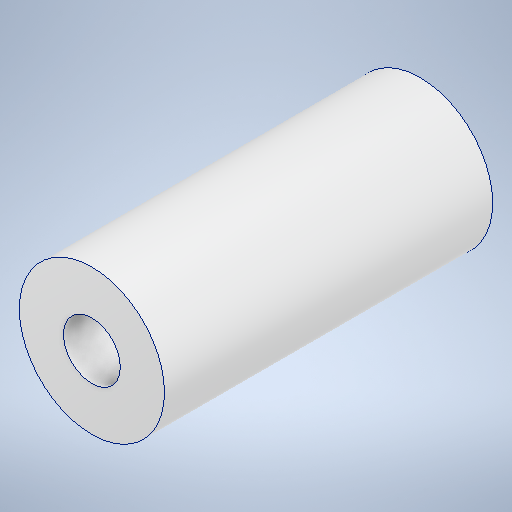
# Autodesk Inventor part: 10-32 0.5 1.131 Inch Stand Off
Saved by Autodesk Inventor 2025.1 (Build 291241020, 241B)
## iProperties
Created: 2024-10-06
Part Number: 10-32 0.5 1.131 Inch Stand Off
Material: Aluminum 6061
Document SubType Name: Modeling
Designer: xmand
Density: 2.7 g/cm^3
Appearance: Aluminum - Flat
Author: xmand
Autodesk Inventor part; units mm, degrees
ref_plane "YZ Plane" through (0, 0, 0) normal (1, 0, 0) x (0, 1, 0)
ref_plane "XZ Plane" through (0, 0, 0) normal (0, 1, 0) x (-1, 0, 0)
ref_plane "XY Plane" through (0, 0, 0) normal (0, 0, 1) x (1, 0, 0)
sketch "Sketch1" plane through (0, 0, 0) normal (0, 0, 1) x (1, 0, 0)
  circle A0 centre (0, 0) radius 2.4892
  circle A1 centre (0, 0) radius 6.35
  dimension "d0" = 4.9784
  dimension "d1" = 12.7
  constraints: 2 centre point, 2 coincident
  measures "d0" diameter of A0
  measures "d1" diameter of A1
extrude "Extrusion1" add sketch "Sketch1" along normal mid plane 28.7274
body "Solid1"
